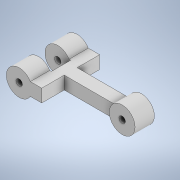
# Autodesk Inventor part: Phalalnge_28mm
Saved by Autodesk Inventor 2021 (Build 250183000, 183)
## iProperties
Created: 2022-08-29
Part Number: Phalalnge_28mm
Material: Generic
Document SubType Name: Modeling
Designer: alyn649
Density: 1 g/cm^3
Appearance: Default
Author: alyn649
Autodesk Inventor part; units mm, degrees
ref_plane "YZ Plane" through (0, 0, 0) normal (1, 0, 0) x (0, 1, 0)
ref_plane "XZ Plane" through (0, 0, 0) normal (0, 1, 0) x (-1, 0, 0)
ref_plane "XY Plane" through (0, 0, 0) normal (0, 0, 1) x (1, 0, 0)
sketch "Sketch1" plane through (0, 0, 0) normal (0, 0, 1) x (1, 0, 0)
  circle A0 centre (-13, 0) radius 1
  circle A1 centre (13, 0) radius 1
  circle A2 centre (-13, 0) radius 4
  circle A3 centre (13, 0) radius 4
  point P0 (0, 0)
  dimension "d0" = 2
  dimension "d1" = 2
  dimension "d3" = 26
  dimension "d4" = 13
  dimension "d5" = 8
  dimension "d6" = 8
  constraints: 4 centre point, 2 coincident, 2 horizontal alignment
  measures "d0" diameter of A0
  measures "d1" diameter of A1
  measures "d3" distance of A1.centre A0.centre
  measures "d4" distance of point (0, 0) A0.centre
  measures "d5" diameter of A2
  measures "d6" diameter of A3
extrude "Extrusion1" add sketch "Sketch1" against normal mid plane 18
sketch "Sketch2" plane through (0, 0, 0) normal (0, 0, 1) x (1, 0, 0)
  circle A0 centre (-13, 0) radius 4 projected
  circle A1 centre (-13, 0) radius 1 projected
  point P0 (0, 0)
extrude "Extrusion2" cut sketch "Sketch2" against normal mid plane 6
sketch "Sketch3" plane through (-13, 0, -3) normal (0, 0, 1) x (1, 0, 0)
  circle A0 centre (26, 0) radius 4 projected
  circle A1 centre (26, 0) radius 4 projected
  circle A2 centre (26, 0) radius 1 projected
  point P0 (13, 0)
extrude "Extrusion3" cut sketch "Sketch3" against normal blind 6
mirror "Mirror1" about plane through (0, 0, 0) normal (0, 0, 1) of "Extrusion3"
sketch "Sketch6" plane through (0, 0, 0) normal (0, 1, 0) x (-1, 0, 0)
  line L0 (-9, -3) -> (-12, -3) construction
  line L1 (-12, -3) -> (-12, 3) construction
  line L2 (-12, 3) -> (-9, 3) construction
  line L3 (-9, 3) -> (-9, -3) construction
  line L4 (-14, -3) -> (-17, -3) construction
  line L5 (-17, -3) -> (-17, 3) construction
  line L6 (-17, 3) -> (-14, 3) construction
  line L7 (-14, 3) -> (-14, -3) construction
  line L8 (9, 9) -> (12, 9) construction
  line L9 (12, 9) -> (12, 3) construction
  line L10 (12, 3) -> (9, 3) construction
  line L11 (9, 3) -> (9, 9) construction
  line L12 (14, 9) -> (17, 9) construction
  line L13 (17, 9) -> (17, 3) construction
  line L14 (17, 3) -> (14, 3) construction
  line L15 (14, 3) -> (14, 9) construction
  line L16 (17, -9) -> (14, -9) construction
  line L17 (14, -9) -> (14, -3) construction
  line L18 (14, -3) -> (17, -3) construction
  line L19 (17, -3) -> (17, -9) construction
  line L20 (12, -9) -> (9, -9) construction
  line L21 (9, -9) -> (9, -3) construction
  line L22 (9, -3) -> (12, -3) construction
  line L23 (12, -3) -> (12, -9) construction
  line L24 (9, -9) -> (17, -9) construction
  line L25 (9, -9) -> (6, -9)
  line L26 (6, -9) -> (6, -2)
  line L27 (6, -2) -> (-9, -2)
  line L28 (-9, 3) -> (-9, -3) construction
  line L29 (-9, 2) -> (6, 2)
  line L30 (6, 2) -> (6, 9)
  line L31 (6, 9) -> (9, 9)
  line L32 (9, -3) -> (17, -3) construction
  line L33 (9, -3) -> (9, 3)
  line L34 (-9, -2) -> (-12, -2)
  line L35 (-12, -3) -> (-12, 3) projected
  line L36 (-9, 2) -> (-12, 2)
  line L37 (9, -9) -> (12, -9)
  line L38 (12, -3) -> (9, -3)
  line L39 (14, -3) -> (12, -3) projected
  line L40 (12, -3) -> (12, -9)
  line L41 (12, -9) -> (12, -3) projected
  line L42 (12, 3) -> (14, 3) projected
  line L43 (17, 3) -> (9, 3) projected
  line L44 (12, 3) -> (9, 3)
  line L45 (12, 9) -> (14, 9) projected
  line L46 (12, 3) -> (12, 9)
  line L47 (17, 9) -> (9, 9) projected
  line L48 (12, 9) -> (9, 9)
  point P0 (0, 0)
  dimension "d16" = 3
  dimension "d17" = 4
  dimension "d18" = 2
  constraints: 30 end point, 6 perpendicular, 6 point on line, 3 collinear, 3 parallel, 1 horizontal, 1 vertical
  measures "d16" distance between parallel lines of L26 L21
  measures "d17" distance between parallel lines of L29 L27
  measures "d18" distance from line of point (0, 0) L27
extrude "Extrusion4" add sketch "Sketch6" against normal mid plane 4
sketch "Sketch7" plane through (-9, -2, -3) normal (-1, 0, 0) x (0, 0, 1)
  circle A0 centre (3, 2) radius 1
  dimension "d21" = 2
  constraints: 1 centre point, 1 coincident
  measures "d21" diameter of A0
extrude "Extrusion5" cut sketch "Sketch7" against normal blind 20
chamfer "Chamfer1" distance 1 angle 45 1 edges at (-9, 0, -1)
equation "\"d4\" = 0.5 * d3"
equation "\"d6\" = d5"
equation "\"d18\" = 0.5 * d17"
body "Solid1"
